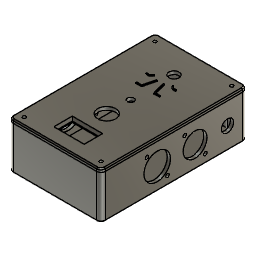
CableTester (Autodesk Fusion 360 design; units mm, degrees)
Autodesk Fusion 360 part; units mm, degrees
note: some values were not read from the file. Set by a fixed rule: which face or edge a step refers to.
sketch "Sketch1" plane through (0, 0, 0) normal (0, 0, 1) x (1, 0, 0) in component "Case"
  line L0 (0, 0) -> (85, 0)
  line L1 (85, 0) -> (85, 135)
  line L2 (85, 135) -> (0, 135)
  line L3 (0, 135) -> (0, 0)
  dimension "d1" = 85
  dimension "d2" = 135
  constraint horizontal L0
  constraint vertical L1
  constraint horizontal L2
  constraint vertical L3
  constraint coincident L0.start L3.end
  measures "d1" distance of L0.start L0.end
  measures "d2" distance of L0.start L2.end
extrude "Extrude1" add sketch "Sketch1" along normal blind 40 makes body 1 in component "Case"
shell "Shell1" thickness 3 removed faces 1 at (28.3333, 90, 40) on bodies 1 in component "Case"
sketch "Sketch2" plane through (0, 0, 40) normal (0, 0, 1) x (-1, 0, 0) in component "Case"
  line L0 (-3, -132) -> (-82, -132)
  line L1 (-82, -132) -> (-82, -3)
  line L2 (-82, -3) -> (-3, -3)
  line L3 (-3, -3) -> (-3, -132)
  line L4 (0, -135) -> (0, 0)
  line L5 (0, 0) -> (-85, 0)
  line L6 (-85, 0) -> (-85, -135)
  line L7 (-85, -135) -> (0, -135)
  line L8 (-3, -3) -> (-82, -82) construction
  line L9 (-3, -3) -> (129.9361, -3) construction
  line L10 (-82, -3) -> (-3, -82) construction
  line L11 (-3, -132) -> (-82, -53) construction
  line L12 (-82, -132) -> (-3, -53) construction
  circle A0 centre (-7, -7) radius 4
  circle A1 centre (-78, -7) radius 4
  circle A2 centre (-7, -128) radius 4
  circle A3 centre (-78, -128) radius 4
  line L13 (-11, -7) -> (-11, -3)
  line L14 (-3, -11) -> (-7, -11)
  line L15 (-3, -124) -> (-7, -124)
  line L16 (-11, -132) -> (-11, -128)
  line L17 (-74, -132) -> (-74, -128)
  line L18 (-82, -124) -> (-78, -124)
  line L19 (-74, -3) -> (-74, -7)
  line L20 (-82, -11) -> (-78, -11)
  circle A4 centre (-7, -7) radius 1.5
  circle A5 centre (-78, -7) radius 1.5
  circle A6 centre (-7, -128) radius 1.5
  circle A7 centre (-78, -128) radius 1.5
  dimension "d6" = 135
  dimension "d7" = 90
  dimension "d8" = 90
  dimension "d9" = 8
  dimension "d10" = 8
  dimension "d11" = 8
  dimension "d12" = 8
  dimension "d13" = 3
  dimension "d14" = 3
  dimension "d15" = 3
  dimension "d16" = 3
  constraint horizontal L9
  constraint coincident L2.end L3.start
  constraint coincident L1 L8.end
  constraint coincident L1.end L2.start
  constraint coincident L3 L10.end
  constraint coincident L0.start L3.end
  constraint coincident L1 L11.end
  constraint perpendicular L8 L11
  constraint coincident L0.end L1.start
  constraint coincident L3 L12.end
  constraint coincident L8 A0.centre
  constraint tangent L2 A0
  constraint coincident L10 A1.centre
  constraint coincident L11 A2.centre
  constraint coincident L12 A3.centre
  constraint tangent L0 A2
  constraint tangent L0 A3
  constraint tangent L2 A1
  constraint coincident A0 L13.start
  constraint coincident L2 L13.end
  constraint perpendicular L2 L13
  constraint tangent A0 L13
  constraint coincident L3 L14.start
  constraint coincident A0 L14.end
  constraint perpendicular L3 L14
  constraint tangent A0 L14
  constraint coincident L3 L15.start
  constraint coincident A2 L15.end
  constraint perpendicular L3 L15
  constraint coincident L0 L16.start
  constraint coincident A2 L16.end
  constraint perpendicular L0 L16
  constraint tangent A2 L16
  constraint tangent A2 L15
  constraint coincident L0 L17.start
  constraint coincident A3 L17.end
  constraint perpendicular L0 L17
  constraint coincident L1 L18.start
  constraint coincident A3 L18.end
  constraint perpendicular L1 L18
  constraint tangent A3 L17
  constraint tangent A3 L18
  constraint coincident L2 L19.start
  constraint coincident A1 L19.end
  constraint perpendicular L2 L19
  constraint coincident L1 L20.start
  constraint coincident A1 L20.end
  constraint perpendicular L1 L20
  constraint tangent A1 L20
  constraint tangent A1 L19
  constraint concentric A0 A4
  constraint concentric A1 A5
  constraint concentric A2 A6
  constraint concentric A3 A7
  measures "d6" angle of L8 L9
  measures "d7" angle of L8 L10
  measures "d8" angle of L11 L12
  measures "d9" diameter of A0
  measures "d10" diameter of A1
  measures "d11" diameter of A2
  measures "d12" diameter of A3
  measures "d13" diameter of A4
  measures "d14" diameter of A5
  measures "d15" diameter of A6
  measures "d16" diameter of A7
extrude "Extrude2" add sketch "Sketch2" against normal up to surface (40 mm away) contours L0 A2 L16 | L0 A3 L17 | L0 L3 A2 | A2 | L0 L1 A3 | A3 | L3 A2 L15 | L1 A3 L18 | L3 A0 L14 | L1 A1 L20 | L2 L3 A0 | A0 | L1 L2 A1 | A1 | L2 A0 L13 | L2 A1 L19 bodies 1 in component "Case"
sketch "Sketch3" plane through (0, 0, 40) normal (0, 0, 1) x (-1, 0, 0) in component "Case"
  line L0 (0, 0) -> (-85, 0)
  line L1 (-85, 0) -> (-85, -135)
  line L2 (-85, -135) -> (0, -135)
  line L3 (0, -135) -> (0, 0)
  point P0 (-85, -135)
  constraint horizontal L0
  constraint vertical L1
  constraint horizontal L2
  constraint vertical L3
  constraint coincident P0 L1.end
  constraint coincident L0.start L3.end
extrude "Extrude3" add sketch "Sketch3" along normal blind 3 separate body makes body 2 in component "Case"
sketch "Sketch4" plane through (85, 0, 0) normal (1, 0, 0) x (0, 1, 0) in component "Case"
  line L0 (0, 0) -> (135, 0)
  line L1 (135, 0) -> (135, 40)
  line L2 (135, 40) -> (0, 40)
  line L3 (0, 40) -> (0, 0)
  line L4 (0, 20) -> (135, 20) construction
  circle A0 centre (117, 20) radius 5.65
  circle A1 centre (87, 20) radius 11
  circle A2 centre (52, 20) radius 12.25
  line L5 (52, 20) -> (52, 0) construction
  line L6 (0, 8) -> (135, 8) construction
  line L7 (0, 32) -> (135, 32) construction
  line L8 (61.5, 8) -> (61.5, 32) construction
  line L9 (42.5, 8) -> (42.5, 32) construction
  circle A3 centre (42.5, 32) radius 1.6
  circle A4 centre (61.5, 8) radius 1.6
  circle A5 centre (42.5, 8) radius 1.6
  circle A6 centre (61.5, 32) radius 1.6
  line L10 (77.5, 32) -> (77.5, 8) construction
  line L11 (96.5, 32) -> (96.5, 8) construction
  line L12 (87, 20) -> (87, 8) construction
  circle A7 centre (77.5, 8) radius 1.6
  circle A8 centre (96.5, 32) radius 1.6
  circle A9 centre (77.5, 32) radius 1.6
  circle A10 centre (96.5, 8) radius 1.6
  dimension "d22" = 11.3
  dimension "d23" = 22
  dimension "d24" = 24.5
  dimension "d25" = 24
  dimension "d26" = 19
  dimension "d27" = 3.2
  dimension "d28" = 3.2
  dimension "d29" = 3.2
  dimension "d30" = 3.2
  dimension "d31" = 19
  dimension "d32" = 3.2
  dimension "d33" = 3.2
  dimension "d34" = 3.2
  dimension "d35" = 3.2
  dimension "d36" = 18
  dimension "d37" = 30
  dimension "d38" = 35
  constraint midpoint L3 L4.start
  constraint midpoint L1 L4.end
  constraint coincident L4 A0.centre
  constraint coincident L4 A1.centre
  constraint coincident L4 A2.centre
  constraint coincident A2.centre L5.start
  constraint coincident L0 L5.end
  constraint perpendicular L0 L5
  constraint coincident L3 L6.start
  constraint coincident L1 L6.end
  constraint perpendicular L1 L6
  constraint coincident L3 L7.start
  constraint coincident L1 L7.end
  constraint perpendicular L1 L7
  constraint symmetric L4 L6 L7
  constraint coincident L6 L8.start
  constraint coincident L7 L8.end
  constraint perpendicular L7 L8
  constraint coincident L6 L9.start
  constraint coincident L7 L9.end
  constraint perpendicular L7 L9
  constraint symmetric L5 L8 L9
  constraint coincident L9.end A3.centre
  constraint coincident L8.start A4.centre
  constraint coincident L9.start A5.centre
  constraint coincident L8.end A6.centre
  constraint coincident L7 L10.start
  constraint coincident L6 L10.end
  constraint perpendicular L6 L10
  constraint coincident L7 L11.start
  constraint coincident L6 L11.end
  constraint perpendicular L6 L11
  constraint coincident A1.centre L12.start
  constraint coincident L6 L12.end
  constraint perpendicular L6 L12
  constraint symmetric L10 L11 L12
  constraint coincident L10.end A7.centre
  constraint coincident L11.start A8.centre
  constraint coincident L10.start A9.centre
  constraint coincident L11.end A10.centre
  measures "d22" diameter of A0
  measures "d23" diameter of A1
  measures "d24" diameter of A2
  measures "d25" distance of L6 L7
  measures "d26" distance of L8 L9
  measures "d27" diameter of A3
  measures "d28" diameter of A4
  measures "d29" diameter of A5
  measures "d30" diameter of A6
  measures "d31" distance of L10 L11
  measures "d32" diameter of A7
  measures "d33" diameter of A8
  measures "d34" diameter of A9
  measures "d35" diameter of A10
  measures "d36" distance of L1 A0.centre
  measures "d37" distance of A0.centre L12
  measures "d38" distance of L5 L12
extrude "Extrude4" cut sketch "Sketch4" against normal up to surface (85 mm away) contours A0 | A1 | A2 bodies 1 in component "Case"
extrude "Extrude5" cut sketch "Sketch4" against normal up to surface (85 mm away) contours A5 | A6 | A7 | A8 bodies 1 in component "Case"
extrude "Extrude6" add sketch "Sketch4" against normal up to surface (3 mm away) contours A5 | A6 | A7 | A8 bodies 1 in component "Case"
extrude "Extrude7" cut sketch "Sketch4" against normal up to surface (3 mm away) contours A3 | A4 | A9 | A10 bodies 1 in component "Case"
sketch "Sketch5" plane through (0, 0, 43) normal (0, 0, 1) x (-1, 0, 0) in component "Case"
  line L0 (0, -135) -> (0, 0)
  line L1 (0, 0) -> (-85, 0)
  line L2 (-85, 0) -> (-85, -135)
  line L3 (-85, -135) -> (0, -135)
  line L4 (-42.5, -135) -> (-42.5, 0) construction
  circle A0 centre (-42.5, -70) radius 3
  circle A1 centre (-42.5, -110) radius 4.65
  line L5 (-30.5, -28) -> (-54.5, -28)
  line L6 (-54.5, -28) -> (-54.5, -15)
  line L7 (-54.5, -15) -> (-30.5, -15)
  line L8 (-30.5, -15) -> (-30.5, -28)
  circle A2 centre (-42.5, -47.8462) radius 8.25
  circle A3 centre (-42.5, -110) radius 12.75 construction
  line L9 (-42.5, -110) -> (-53.2061, -98.1097) construction
  line L10 (-42.5, -110) -> (-48.4565, -86.1097) construction
  line L11 (-53.2061, -98.1097) -> (-56.2061, -98.1097) construction
  line L12 (-48.4565, -86.1097) -> (-53.4565, -86.1097) construction
  line L13 (-42.1284, -109.6654) -> (-52.9835, -97.6097)
  line L14 (-52.9835, -97.6097) -> (-56.2061, -97.6097)
  line L15 (-42.8716, -110.3346) -> (-53.4287, -98.6097)
  line L16 (-53.4287, -98.6097) -> (-56.2061, -98.6097)
  line L17 (-42.0149, -109.879) -> (-48.0659, -85.6097)
  line L18 (-48.0659, -85.6097) -> (-53.4565, -85.6097)
  line L19 (-42.9851, -110.121) -> (-48.8472, -86.6097)
  line L20 (-48.8472, -86.6097) -> (-53.4565, -86.6097)
  line L21 (-56.2061, -98.6097) -> (-56.2061, -97.6097)
  line L22 (-53.4565, -86.6097) -> (-53.4565, -85.6097)
  line L23 (-51.3964, -100.8668) -> (-50.6533, -100.1976)
  line L24 (-46.0673, -97.7592) -> (-45.097, -97.5173)
  line L25 (-42.8716, -109.6654) -> (-32.0165, -97.6097)
  line L26 (-32.0165, -97.6097) -> (-28.7939, -97.6097)
  line L27 (-28.7939, -98.6097) -> (-28.7939, -97.6097)
  line L28 (-31.5713, -98.6097) -> (-28.7939, -98.6097)
  line L29 (-42.1284, -110.3346) -> (-31.5713, -98.6097)
  line L30 (-42.5, -110) -> (-31.7939, -98.1097) construction
  line L31 (-33.6036, -100.8668) -> (-34.3467, -100.1976)
  line L32 (-38.9327, -97.7592) -> (-39.903, -97.5173)
  line L33 (-36.1528, -86.6097) -> (-31.5435, -86.6097)
  line L34 (-31.5435, -86.6097) -> (-31.5435, -85.6097)
  line L35 (-36.9341, -85.6097) -> (-31.5435, -85.6097)
  line L36 (-42.9851, -109.879) -> (-36.9341, -85.6097)
  line L37 (-42.0149, -110.121) -> (-36.1528, -86.6097)
  line L38 (-42.5, -110) -> (-36.5435, -86.1097) construction
  dimension "d47" = 6
  dimension "d48" = 65
  dimension "d49" = 9.3
  dimension "d50" = 25
  dimension "d58" = 24
  dimension "d59" = 13
  dimension "d60" = 15
  dimension "d62" = 16.5
  dimension "d63" = 25.5
  dimension "d66" = 42
  dimension "d67" = 14
  dimension "d68" = 3
  dimension "d69" = 5
  dimension "d70" = 12
  dimension "d71" = 16
  dimension "d72" = 0.5
  dimension "d73" = -0.5
  dimension "d74" = 0.5
  dimension "d75" = -0.5
  dimension "d76" = 28
  constraint midpoint L3 L4.start
  constraint midpoint L1 L4.end
  constraint coincident L4 A0.centre
  constraint coincident L4 A1.centre
  constraint horizontal L5
  constraint vertical L6
  constraint horizontal L7
  constraint vertical L8
  constraint symmetric L4 L6 L8
  constraint coincident L4 A2.centre
  constraint concentric A1 A3
  constraint coincident A1.centre A3.centre
  constraint horizontal L11
  constraint horizontal L12
  constraint perpendicular L14 L21
  constraint perpendicular L18 L22
  constraint coincident A3 L23.start
  constraint coincident L15 L23.start
  constraint coincident A3 L23.end
  constraint coincident L13 L23.end
  constraint coincident A3 L24.start
  constraint coincident L19 L24.start
  constraint coincident L17 L24.end
  constraint coincident A3 L24.end
  constraint symmetric L4 A1.centre A3.centre
  constraint symmetric L4 L9.end L30.end
  constraint symmetric L4 L10.end L38.end
  constraint symmetric L4 L13.start L25.start
  constraint symmetric L4 L13.end L25.end
  constraint symmetric L4 L14.end L26.end
  constraint symmetric L4 L15.start L29.start
  constraint symmetric L4 L15.end L28.start
  constraint symmetric L4 L16.end L27.start
  constraint symmetric L4 L17.start L36.start
  constraint symmetric L4 L17.end L35.start
  constraint symmetric L4 L18.end L34.end
  constraint symmetric L4 L19.start L37.start
  constraint symmetric L4 L19.end L33.start
  constraint symmetric L4 L20.end L33.end
  constraint symmetric L4 L23.start L31.start
  constraint symmetric L4 L23.end L31.end
  constraint symmetric L4 L24.start L32.start
  constraint symmetric L4 L24.end L32.end
  measures "d47" diameter of A0
  measures "d48" distance of L3 A0.centre
  measures "d49" diameter of A1
  measures "d50" distance of L3 A1.centre
  measures "d58" distance of L6.end L7.end
  measures "d59" distance of L5.end L6.end
  measures "d60" distance of L1 L7
  measures "d62" diameter of A2
  measures "d63" diameter of A3
  measures "d66" angle of L4 L9
  measures "d67" angle of L4 L10
  measures "d68" distance of L9.end L11.end
  measures "d69" distance of L10.end L12.end
  measures "d70" distance of L11 L12
  measures "d71" distance of A1.centre L9.end
  measures "d76" angle of L10 L38
extrude "Extrude10" add sketch "Sketch5" along normal blind 0.5 contours L25 L26 L27 L28 L29 L31 | L13 L14 L15 L16 L21 L23 | L32 L33 L34 L35 L36 L37 | L17 L18 L19 L20 L22 L24 bodies 2 in component "Case"
extrude "Extrude8" cut sketch "Sketch5" against normal up to surface (3 mm away) contours A0 | A1 L13 L25 | A1 L25 L37 | A1 L13 L19 | A1 L17 L25 L36 L37 | A1 L13 L17 L19 L36 | A1 L17 L36 | L13 L17 L25 L36 | L5 L6 L7 L8 | A2 bodies 2 in component "Case"
extrude "Extrude9" cut sketch "Sketch2" along normal up to surface (3 mm away) contours A4 | A5 | A6 | A7 bodies 2 in component "Case"
fillet "Fillet1" radius 4 8 edges at (85, 135, 20) (0, 135, 20) (0, 0, 20) (85, 0, 20) (85, 135, 41.5) (0, 135, 41.5) (0, 0, 41.5) (85, 0, 41.5) on bodies 1 2 in component "Case"
chamfer "Chamfer1" distance 1 angle 45 16 edges at (42.5, 135, 0) (1.1716, 133.8284, 0) (0, 67.5, 0) (1.1716, 1.1716, 0) (42.5, 0, 0) (83.8284, 1.1716, 0) (85, 67.5, 0) (83.8284, 133.8284, 0) (42.5, 135, 43) (1.1716, 133.8284, 43) (0, 67.5, 43) (1.1716, 1.1716, 43) (42.5, 0, 43) (83.8284, 1.1716, 43) (85, 67.5, 43) (83.8284, 133.8284, 43) on bodies 1 2 in component "Case"
chamfer "Chamfer2" distance 2 angle 45 4 edges at (30.5, 21.5, 43) (42.5, 15, 43) (54.5, 21.5, 43) (42.5, 28, 43) on bodies 2 in component "Case"
component "Case" placed x (1, 0, 0) y (0, 1, 0) z (0, 0, 1) at (0, 0, 0)
equation "d10 = d9"
equation "d11 = d9"
equation "d12 = d9"
equation "d14 = d13"
equation "d15 = d13"
equation "d16 = d13"
equation "d67 = d66 / 3"
